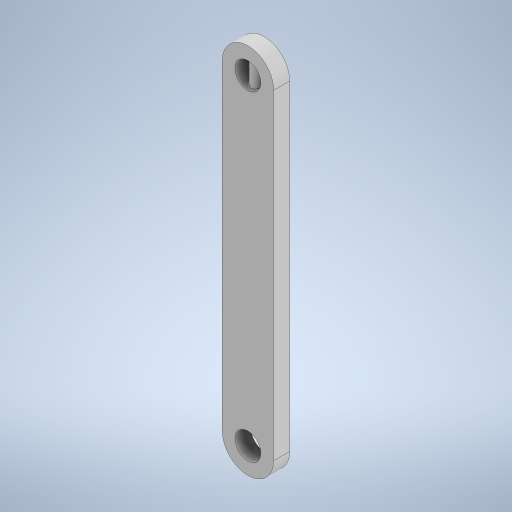
# Autodesk Inventor part: HUDSON 1-14 LEAFSPRING HANGER-1
Saved by Autodesk Inventor 2024.2 (Build 282272000, 272)
## iProperties
Created: 2024-10-08
Part Number: HUDSON 1-14 LEAFSPRING HANGER-1
Material: Generic
Document SubType Name: Modeling
Designer: Jimena Brenes
Density: 1 g/cm^3
Appearance: Default
Author: Jimena Brenes
Autodesk Inventor part; units mm, degrees
ref_plane "XZ Plane" through (0, 0, 0) normal (0, 1, 0) x (-1, 0, 0)
ref_plane "XY Plane" through (0, 0, 0) normal (0, 0, 1) x (1, 0, 0)
sketch "Sketch1" plane through (0, 0, 0) normal (0, 0, 1) x (1, 0, 0)
  arc A0 (4, 0) -> (-4, 0) centre (0, 0) ccw
  circle A1 centre (0, 0) radius 2
  line L0 (0, -2) -> (0, 2)
  line L1 (-0.75, -1.854) -> (-0.75, 1.854)
  arc A2 (-4, -50) -> (4, -50) centre (0, -50) ccw
  circle A3 centre (0, -50) radius 2
  line L2 (-4, 0) -> (-4, -50)
  line L3 (4, 0) -> (4, -50)
  dimension "d1" = 4
  dimension "d2" = 8
  dimension "d3" = 1.5
  dimension "d4" = 8
  dimension "d5" = 4
  dimension "d6" = 50
  constraints: 8 end point, 7 point on circle, 4 centre point, 4 coincident, 3 tangent, 3 vertical, 1 midpoint, 1 parallel
  measures "d1" diameter of A1
  measures "d2" diameter of A0
  measures "d3" diameter of L1 L0
  measures "d4" diameter of A2
  measures "d5" diameter of A3
  measures "d6" distance of A2.centre point (0, 0)
extrude "Extrusion1" add sketch "Sketch1" along normal blind 2.5
ref_plane "Work Plane1" through (0, 0, 0) normal (1, 0, 0) x (0, 1, 0)
sketch "Sketch2" plane through (0, 0, 0) normal (1, 0, 0) x (0, 1, 0)
  line L0 (-2, 1.25) -> (2, 1.25)
  line L1 (-2, 0) -> (2, 0) projected
  line L2 (2, 2) -> (-2, 2)
  line L3 (2, 2) -> (2, 1.25)
  line L4 (-2, 2) -> (-2, 1.25)
  point P0 (0, 0)
  dimension "d11" = 1.25
  dimension "d12" = 1.5
  dimension "d13" = 4
  constraints: 8 end point, 1 horizontal, 1 parallel, 1 vertical
  measures "d11" distance between parallel lines of L1 L0
  measures "d12" diameter of L2 L0
  measures "d13" distance between parallel lines of L4 L3
revolve "Revolution2" add sketch "Sketch2" angle 360 about axis through (0, -2, 1.25) along (0, 1, 0)
body "Solid1"
